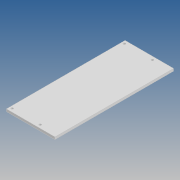
# Autodesk Inventor part: KB33-046-004-002 - Передняя пластина
Saved by Autodesk Inventor 2020 (Build 240168000, 168)
## iProperties
Created: 2021-06-25
Part Number: KB33-046-004-002 - Передняя пластина
Material: Типовые
Document SubType Name: Modeling
Designer: Петров Иван
Mass: 67.2513 g
Surface Area: 360.999 cm^2
Volume: 67.2513 cm^3
Density: 1 g/cm^3
Appearance: По умолчанию
Author: Петров Иван
Autodesk Inventor part; units mm, degrees
ref_plane "YZ Plane" through (0, 0, 0) normal (1, 0, 0) x (0, 1, 0)
ref_plane "XZ Plane" through (0, 0, 0) normal (0, 1, 0) x (-1, 0, 0)
ref_plane "XY Plane" through (0, 0, 0) normal (0, 0, 1) x (1, 0, 0)
sketch "Эскиз1" plane through (0, 0, 0) normal (0, 1, 0) x (-1, 0, 0)
  line L0 (-2.6795, -19) -> (83.0251, -19)
  line L1 (-2.6795, 184) -> (83.0251, 184)
  circle A0 centre (30.7479, 178.5) radius 1.85
  circle A1 centre (78.7479, 178.5) radius 1.85
  circle A2 centre (78.7479, -13.5) radius 1.85
  circle A3 centre (30.7479, -13.5) radius 1.85
  line L2 (83.0251, 184) -> (-2.6795, 184)
  line L3 (-2.6795, 184) -> (-2.6795, -19)
  line L4 (-2.6795, -19) -> (83.0251, -19)
  line L5 (83.0251, -19) -> (83.0251, 184)
  point P0 (0, 0)
  point P1 (83.0251, -19)
  constraints: 12 end point, 4 centre point, 2 parallel, 1 horizontal, 1 perpendicular
extrude "Выдавливание1" add sketch "Эскиз1" along normal blind 4
thicken "Толщина1" operation add thickness 2.671 both sides no extend neighbours yes toward (-1, 0, 0) faces at (2.6795, 1.3333, 116.3333)
